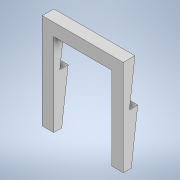
# Autodesk Inventor part: gasketForVacuum
Saved by Autodesk Inventor 2022.1 (Build 261234020, 234B)
## iProperties
Created: 2020-08-29
Part Number: gasketForVacuum
Material: Generic
Document SubType Name: Modeling
Designer: robst
Density: 1 g/cm^3
Appearance: Default
Author: robst
Autodesk Inventor part; units mm, degrees
ref_plane "YZ Plane" through (0, 0, 0) normal (1, 0, 0) x (0, 1, 0)
ref_plane "XZ Plane" through (0, 0, 0) normal (0, 1, 0) x (-1, 0, 0)
ref_plane "XY Plane" through (0, 0, 0) normal (0, 0, 1) x (1, 0, 0)
sketch "Sketch4" plane through (0, 0, 0) normal (1, 0, 0) x (0, 1, 0)
  line L0 (0, 0) -> (0, -12.7)
  line L1 (0, -12.7) -> (-101.6, 0)
  line L2 (-101.6, 0) -> (-101.6, -12.7)
  line L3 (-101.6, -12.7) -> (-203.2, 0)
  line L4 (-203.2, 0) -> (-203.2, -12.7)
  line L5 (-203.2, -12.7) -> (-304.8, 0)
  line L6 (-34.29, -8.4137) -> (-34.29, 9.3662)
  line L7 (-34.29, 9.3662) -> (-180.34, 9.3662)
  line L8 (-180.34, 9.3662) -> (-180.34, -2.8575)
  dimension "d28" = 12.7
  dimension "d29" = 101.6
  dimension "d30" = 101.6
  dimension "d31" = 12.7
  dimension "d32" = 101.6
  dimension "d33" = 146.05
  dimension "d34" = 17.78
  dimension "d35" = 67.31
  constraints: 18 end point, 5 vertical, 2 point on line, 1 perpendicular
  measures "d28" distance of L0.start L0.end
  measures "d29" distance of L1.end L0.start
  measures "d30" distance of L3.end L1.end
  measures "d31" distance of L3.end L4.end
  measures "d32" distance of L5.end L3.end
  measures "d33" distance of L6.end L7.end
  measures "d34" distance of L6.start L6.end
  measures "d35" distance from line of L1.end L6
extrude "Extrusion6" add sketch "Sketch4" along normal mid plane 123.825
sketch "Sketch6" plane through (-61.9125, -180.34, 9.3662) normal (0, 0, 1) x (1, 0, 0)
  line L0 (0, 0) -> (123.825, 0) construction
  line L1 (61.9125, 0) -> (61.9125, 146.05) construction
  line L2 (0, 146.05) -> (123.825, 146.05) construction
  line L3 (17.4625, 0) -> (106.3625, 0)
  line L4 (106.3625, 0) -> (106.3625, 127)
  line L5 (106.3625, 127) -> (17.4625, 127)
  line L6 (17.4625, 127) -> (17.4625, 0)
  line L7 (17.4625, 0) -> (106.3625, 127) construction
  line L8 (106.3625, 0) -> (17.4625, 127) construction
  line L9 (0, 78.74) -> (123.825, 78.74) projected
  point P0 (61.9125, 180.34)
  point P1 (61.9125, 63.5)
  dimension "d59" = 127
  dimension "d60" = 88.9
  constraints: 14 end point, 4 midpoint, 3 parallel, 1 collinear, 1 perpendicular, 1 point on line
  measures "d59" distance of L5.end L3.start
  measures "d60" distance of L4.end L5.end
extrude "Extrusion7" cut sketch "Sketch6" against normal through all
equation "\"sidingHeight\" = 101.6"
equation "\"sidingDepth\" = 12.7"
equation "\"radiusOfCurvature\" = 609.6"
equation "\"outsideWidthOfVent\" = 152.4"
equation "\"wallThicknessOfVent\" = 19.05"
equation "\"holeOffset\" = 6.35"
equation "\"ventHole\" = 114.3"
equation "\"ventRadius\" = 6.35"
body "Solid3"
